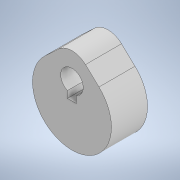
# Autodesk Inventor part: Cam 4
Saved by Autodesk Inventor 2021 (Build 250183000, 183)
## iProperties
Created: 2021-04-12
Part Number: Cam 4
Material: Generic
Document SubType Name: Modeling
Designer: Nabeel Azafer
Density: 1 g/cm^3
Appearance: Default
Author: Nabeel Azafer
Autodesk Inventor part; units mm, degrees
ref_plane "YZ Plane" through (0, 0, 0) normal (1, 0, 0) x (0, 1, 0)
ref_plane "XZ Plane" through (0, 0, 0) normal (0, 1, 0) x (-1, 0, 0)
ref_plane "XY Plane" through (0, 0, 0) normal (0, 0, 1) x (1, 0, 0)
sketch "Sketch1" plane through (0, 0, 0) normal (0, 0, 1) x (1, 0, 0)
  arc A0 (-5.9879, 6.3802) -> (5.9879, 6.3802) centre (0, 0) ccw
  arc A1 (2.994, 9.1901) -> (-2.994, 9.1901) centre (0, 6) ccw
  line L0 (-2.994, 9.1901) -> (-5.9879, 6.3802)
  line L1 (2.994, 9.1901) -> (5.9879, 6.3802)
  circle A2 centre (0, 4.5) radius 2.5
  line L2 (1, 2.2087) -> (-1, 2.2087)
  line L3 (-1, 2.2087) -> (-1, 0.7087)
  line L4 (-1, 0.7087) -> (1, 0.7087)
  line L5 (1, 0.7087) -> (1, 2.2087)
  dimension "d3" = 5
  dimension "d0" = 17.5
  dimension "d1" = 6
  dimension "d2" = 8.75
  dimension "d4" = 4.5
  dimension "d7" = 2
  dimension "d8" = 1.5
  constraints: 12 end point, 4 point on circle, 4 tangent, 2 centre point, 2 parallel, 1 coincident, 1 horizontal, 1 perpendicular, 3 other
  measures "d0" diameter of A0
  measures "d1" distance of point (0, 0) A1.centre
  measures "d2" diameter of A1
  measures "d4" distance of point (0, 0) point (0, 4.5)
  measures "d7" distance of L4.end L3.end
  measures "d8" distance of L3.end L2.end
extrude "Extrusion1" add sketch "Sketch1" along normal blind 8
body "Solid1"
